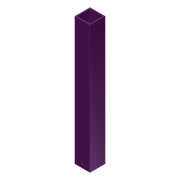
# Autodesk Inventor part: CentralColumn
Saved by Autodesk Inventor 2012 (Build 160160000, 160)
## iProperties
Created: 2013-01-12
Part Number: CentralColumn
Material: Aluminum-6061
Document SubType Name: Modeling
Designer: JesseK
Density: 2.71 g/cm^3
Mass: 706.541 g
Surface Area: 1656.3 cm^2
Volume: 260.716 cm^3
Author: JesseK
Autodesk Inventor part; units mm, degrees
ref_plane "YZ Plane" through (0, 0, 0) normal (1, 0, 0) x (0, 1, 0)
ref_plane "XZ Plane" through (0, 0, 0) normal (0, 1, 0) x (-1, 0, 0)
ref_plane "XY Plane" through (0, 0, 0) normal (0, 0, 1) x (1, 0, 0)
sketch "Sketch1" plane through (0, 0, 0) normal (0, 0, 1) x (1, 0, 0)
  line L0 (0, 0) -> (50.8, 0)
  line L1 (50.8, 0) -> (50.8, 431.8)
  line L2 (50.8, 431.8) -> (0, 431.8)
  line L3 (0, 431.8) -> (0, 0)
  dimension "d0" = 50.8
  dimension "d1" = 431.8
  constraints: 8 end point, 2 parallel, 1 horizontal, 1 perpendicular
  measures "d0" distance of L0.start L0.end
  measures "d1" distance of L2.end L0.start
extrude "Extrusion1" add sketch "Sketch1" along normal blind 50.8
shell "Shell1" thickness 3.175 removed faces 2 at (33.8667, 431.8, 16.9333) at (16.9333, 0, 16.9333)
sketch "Sketch3" plane through (0, 0, 50.8) normal (0, 0, 1) x (1, 0, 0)
  line L0 (50.8, 0) -> (0, 0) projected
  line L1 (50.8, 431.8) -> (50.8, 0) projected
  circle A0 centre (25.4, 9.525) radius 3.175
  dimension "d10" = 9.525
  dimension "d11" = 25.4
  dimension "d12" = 6.35
  constraints: 1 centre point
  measures "d10" distance from line of L0 A0.centre
  measures "d11" distance from line of L1 A0.centre
  measures "d12" diameter of A0
extrude "Extrusion3" cut sketch "Sketch3" against normal through all
body "Solid1"
